Autodesk Fusion 360 part; units mm, degrees
(part 5 of 5)
sketch "Sketch4" plane through (0, 0, 0) normal (0, 0, -1) x (1, 0, 0)
  spline S0 degree 3 poles (245.0152, -3.6397) (245.0152, -3.0095) (244.82, -2.6944) (244.4293, -2.6944) knots -1 -1 -1 -1 0 0 0 0
  spline S1 degree 3 poles (244.2163, -5.1842) (244.7489, -4.6693) (245.0152, -4.1546) (245.0152, -3.6397) knots -1 -1 -1 -1 0 0 0 0
  spline S2 degree 3 poles (243.9766, -3.2536) (243.9766, -3.2625) (244.0565, -3.906) (244.2163, -5.1842) knots -1 -1 -1 -1 0 0 0 0
  spline S3 degree 3 poles (244.4293, -2.6944) (244.1277, -2.6944) (243.9766, -2.8808) (243.9766, -3.2536) knots -1 -1 -1 -1 0 0 0 0
  spline S4 degree 3 poles (271.6477, -6.9285) (271.8784, -6.9285) (272.1314, -6.8752) (272.4066, -6.7687) knots -1 -1 -1 -1 0 0 0 0
  spline S5 degree 3 poles (270.2896, -6.276) (270.6268, -6.711) (271.0795, -6.9285) (271.6477, -6.9285) knots -1 -1 -1 -1 0 0 0 0
  spline S6 degree 3 poles (269.7037, -4.3587) (269.7657, -5.2109) (269.9611, -5.85) (270.2896, -6.276) knots -1 -1 -1 -1 0 0 0 0
  spline S7 degree 3 poles (269.6904, -4.1324) (269.6904, -4.2033) (269.6948, -4.2788) (269.7037, -4.3587) knots -1 -1 -1 -1 0 0 0 0
  spline S8 degree 3 poles (269.9967, -3.0938) (269.7924, -3.3512) (269.6904, -3.6973) (269.6904, -4.1324) knots -1 -1 -1 -1 0 0 0 0
  spline S9 degree 3 poles (270.8089, -2.7077) (270.4804, -2.7077) (270.2097, -2.8365) (269.9967, -3.0938) knots -1 -1 -1 -1 0 0 0 0
  spline S10 degree 3 poles (272.0738, -3.8794) (271.7896, -3.0982) (271.3681, -2.7077) (270.8089, -2.7077) knots -1 -1 -1 -1 0 0 0 0
  line L0 (272.0738, -3.8794) -> (272.4066, -6.7687)
  spline S11 degree 3 poles (249.2375, -3.3867) (249.2375, -3.5998) (249.2951, -4.1546) (249.4106, -5.0511) knots -1 -1 -1 -1 0 0 0 0
  spline S12 degree 3 poles (249.4638, -2.8675) (249.313, -3.0095) (249.2375, -3.1826) (249.2375, -3.3867) knots -1 -1 -1 -1 0 0 0 0
  spline S13 degree 3 poles (250.1162, -2.6677) (249.841, -2.6677) (249.6236, -2.7343) (249.4638, -2.8675) knots -1 -1 -1 -1 0 0 0 0
  spline S14 degree 3 poles (251.2347, -3.2935) (250.9418, -2.8764) (250.5689, -2.6677) (250.1162, -2.6677) knots -1 -1 -1 -1 0 0 0 0
  spline S15 degree 3 poles (251.7673, -5.2641) (251.7673, -4.4563) (251.5898, -3.7995) (251.2347, -3.2935) knots -1 -1 -1 -1 0 0 0 0
  spline S16 degree 3 poles (251.501, -6.3027) (251.6784, -6.0008) (251.7673, -5.6546) (251.7673, -5.2641) knots -1 -1 -1 -1 0 0 0 0
  spline S17 degree 3 poles (250.6755, -6.7554) (251.0483, -6.7554) (251.3235, -6.6045) (251.501, -6.3027) knots -1 -1 -1 -1 0 0 0 0
  spline S18 degree 3 poles (249.5171, -5.85) (249.7834, -6.4536) (250.1695, -6.7554) (250.6755, -6.7554) knots -1 -1 -1 -1 0 0 0 0
  line L1 (249.5171, -5.85) -> (249.4106, -5.0511)
  spline S19 degree 3 poles (270.0499, 0.4346) (270.0499, -0.311) (270.6402, -1.0344) (271.8208, -1.7357) knots -1 -1 -1 -1 0 0 0 0
  spline S20 degree 3 poles (270.2496, 0.9938) (270.1165, 0.8607) (270.0499, 0.6743) (270.0499, 0.4346) knots -1 -1 -1 -1 0 0 0 0
  spline S21 degree 3 poles (270.729, 1.2068) (270.5513, 1.2068) (270.3915, 1.1359) (270.2496, 0.9938) knots -1 -1 -1 -1 0 0 0 0
  spline S22 degree 3 poles (271.5944, 0.2615) (271.5145, 0.8917) (271.226, 1.2068) (270.729, 1.2068) knots -1 -1 -1 -1 0 0 0 0
  line L2 (271.5944, 0.2615) -> (271.8208, -1.7357)
  spline S23 degree 3 poles (254.5822, -2.0872) (254.0928, -2.1577) (253.5454, -2.2239) (253.0284, -2.2637) knots 0.397503 0.397503 0.397503 0.397503 1 1 1 1
  spline S24 degree 3 poles (253.0284, -2.2637) (252.7959, -2.2817) (252.5688, -2.2944) (252.3554, -2.2998) knots 0 0 0 0 0.530693 0.530693 0.530693 0.530693
  spline S25 degree 3 poles (252.3554, -2.2998) (251.6864, -1.7551) (250.829, -1.4827) (249.7834, -1.4827) knots 0.050062 0.050062 0.050062 0.050062 1 1 1 1
  spline S26 degree 3 poles (249.7834, -1.4827) (249.3396, -1.5004) (248.9535, -1.5803) (248.625, -1.7224) knots 0 0 0 0 1 1 1 1
  spline S27 degree 3 poles (248.625, -1.7224) (248.2965, -1.8645) (248.0525, -2.0419) (247.8927, -2.255) knots 0 0 0 0 1 1 1 1
  spline S28 degree 3 poles (247.8927, -2.255) (247.6718, -2.5408) (247.5317, -2.8028) (247.4725, -3.0411) knots 0 0 0 0 0.731862 0.731862 0.731862 0.731862
  spline S29 degree 3 poles (247.4725, -3.0411) (247.287, -3.1929) (247.0989, -3.2785) (246.9137, -3.3116) knots 0.13739 0.13739 0.13739 0.13739 1 1 1 1
  spline S30 degree 3 poles (246.9137, -3.3116) (246.6993, -3.35) (246.4954, -3.3167) (246.3122, -3.2441) knots 0 0 0 0 1 1 1 1
  spline S31 degree 3 poles (246.3122, -3.2441) (246.1226, -3.1688) (245.953, -3.0508) (245.812, -2.9222) knots 0 0 0 0 0.743467 0.743467 0.743467 0.743467
  spline S32 degree 3 poles (245.812, -2.9222) (245.7256, -2.5498) (245.5577, -2.2475) (245.3081, -2.0153) knots 0.346286 0.346286 0.346286 0.346286 1 1 1 1
  spline S33 degree 3 poles (245.3081, -2.0153) (244.9265, -1.6602) (244.4472, -1.4827) (243.8701, -1.4827) knots 0 0 0 0 1 1 1 1
  spline S34 degree 3 poles (243.8701, -1.4827) (243.2932, -1.4827) (242.8715, -1.6602) (242.6052, -2.0153) knots 0 0 0 0 1 1 1 1
  spline S35 degree 3 poles (242.6052, -2.0153) (242.357, -2.3545) (242.2244, -2.7749) (242.2076, -3.2761) knots 0 0 0 0 0.932227 0.932227 0.932227 0.932227
  spline S36 degree 3 poles (242.2076, -3.2761) (241.9882, -3.027) (241.7354, -2.7798) (241.4493, -2.5346) knots 0.616308 0.616308 0.616308 0.616308 1 1 1 1
  spline S37 degree 3 poles (241.4493, -2.5346) (241.0765, -2.224) (240.6327, -1.971) (240.1178, -1.7757) knots 0 0 0 0 1 1 1 1
  spline S38 degree 3 poles (240.1178, -1.7757) (239.6119, -1.5803) (239.0882, -1.4827) (238.5467, -1.4827) knots 0 0 0 0 1 1 1 1
  spline S39 degree 3 poles (238.5467, -1.4827) (237.659, -1.4827) (236.9578, -1.7534) (236.4429, -2.2949) knots 0 0 0 0 1 1 1 1
  spline S40 degree 3 poles (236.4429, -2.2949) (235.8938, -2.8795) (235.6187, -3.6274) (235.6174, -4.5389) knots 0 0 0 0 0.99774 0.99774 0.99774 0.99774
  spline S41 degree 3 poles (235.6174, -4.5389) (235.515, -4.5909) (235.4125, -4.6249) (235.3108, -4.6431) knots 0.526695 0.526695 0.526695 0.526695 1 1 1 1
  spline S42 degree 3 poles (235.3108, -4.6431) (235.0964, -4.6815) (234.8926, -4.6482) (234.7093, -4.5756) knots 0 0 0 0 1 1 1 1
  spline S43 degree 3 poles (234.7093, -4.5756) (234.6486, -4.5514) (234.5899, -4.5229) (234.5335, -4.4911) knots 0 0 0 0 0.23829 0.23829 0.23829 0.23829
  spline S44 degree 3 poles (234.5335, -4.4911) (234.3844, -3.9886) (234.2169, -3.5717) (234.031, -3.2403) knots 0.544726 0.544726 0.544726 0.544726 1 1 1 1
  spline S45 degree 3 poles (234.031, -3.2403) (233.8446, -2.9297) (233.6316, -2.6322) (233.3919, -2.3482) knots 0 0 0 0 1 1 1 1
  spline S46 degree 3 poles (233.3919, -2.3482) (232.8948, -1.7713) (232.198, -1.4827) (231.3015, -1.4827) knots 0 0 0 0 1 1 1 1
  spline S47 degree 3 poles (231.3015, -1.4827) (230.4138, -1.4827) (229.7792, -1.8645) (229.3975, -2.6278) knots 0 0 0 0 1 1 1 1
  spline S48 degree 3 poles (229.3975, -2.6278) (228.9093, -1.8645) (228.1681, -1.4827) (227.1739, -1.4827) knots 0 0 0 0 1 1 1 1
  spline S49 degree 3 poles (227.1739, -1.4827) (226.5348, -1.4827) (226.0377, -1.6648) (225.6827, -2.0286) knots 0 0 0 0 1 1 1 1
  spline S50 degree 3 poles (225.6827, -2.0286) (225.3365, -2.4014) (225.1634, -2.8941) (225.1634, -3.5066) knots 0 0 0 0 1 1 1 1
  spline S51 degree 3 poles (225.1634, -3.5066) (225.1634, -3.5865) (225.1723, -3.7063) (225.19, -3.8661) knots 0 0 0 0 1 1 1 1
  line L3 (225.19, -3.8661) -> (225.6827, -7.6208)
  spline S52 degree 3 poles (225.6827, -7.6208) (224.7329, -8.3043) (224.258, -9.0721) (224.258, -9.9243) knots 0 0 0 0 1 1 1 1
  spline S53 degree 3 poles (224.258, -9.9243) (224.258, -10.4658) (224.4444, -10.8963) (224.8172, -11.2158) knots 0 0 0 0 1 1 1 1
  spline S54 degree 3 poles (224.8172, -11.2158) (225.19, -11.5354) (225.6427, -11.6952) (226.1753, -11.6952) knots 0 0 0 0 1 1 1 1
  spline S55 degree 3 poles (226.1753, -11.6952) (227.3381, -11.6952) (227.9195, -11.1182) (227.9195, -9.9642) knots 0 0 0 0 1 1 1 1
  spline S56 degree 3 poles (227.9195, -9.9642) (227.9195, -9.9465) (227.9151, -9.9243) (227.9062, -9.8977) knots 0 0 0 0 1 1 1 1
  spline S57 degree 3 poles (227.9062, -9.8977) (227.9062, -9.871) (227.9018, -9.8267) (227.8929, -9.7645) knots 0 0 0 0 1 1 1 1
  spline S58 degree 3 poles (227.8929, -9.7645) (227.8929, -9.7113) (227.884, -9.6447) (227.8663, -9.5648) knots 0 0 0 0 1 1 1 1
  spline S59 degree 3 poles (227.8663, -9.5648) (227.8574, -9.4938) (227.8396, -9.3828) (227.813, -9.2319) knots 0 0 0 0 1 1 1 1
  spline S60 degree 3 poles (227.813, -9.2319) (227.7953, -9.081) (227.7731, -8.9124) (227.7464, -8.726) knots 0 0 0 0 1 1 1 1
  spline S61 degree 3 poles (227.7464, -8.726) (227.7198, -8.5484) (227.6843, -8.3088) (227.6399, -8.007) knots 0 0 0 0 1 1 1 1
  spline S62 degree 3 poles (227.6399, -8.007) (227.5955, -7.7052) (227.5467, -7.3767) (227.4935, -7.0217) knots 0 0 0 0 1 1 1 1
  spline S63 degree 3 poles (227.4935, -7.0217) (227.4491, -6.6755) (227.3914, -6.2494) (227.3204, -5.7434) knots 0 0 0 0 1 1 1 1
  spline S64 degree 3 poles (227.3204, -5.7434) (227.2494, -5.2375) (227.1872, -4.807) (227.134, -4.4519) knots 0 0 0 0 1 1 1 1
  spline S65 degree 3 poles (227.134, -4.4519) (227.0807, -4.0968) (227.0541, -3.8394) (227.0541, -3.6797) knots 0 0 0 0 1 1 1 1
  spline S66 degree 3 poles (227.0541, -3.6797) (227.0541, -3.0849) (227.2849, -2.7876) (227.7464, -2.7876) knots 0 0 0 0 1 1 1 1
  spline S67 degree 3 poles (227.7464, -2.7876) (228.3855, -2.7876) (228.7806, -3.369) (228.9314, -4.5318) knots 0 0 0 0 1 1 1 1
  line L4 (228.9314, -4.5318) -> (229.7836, -11.2558)
  spline S68 degree 3 poles (229.7836, -11.2558) (230.0765, -11.3889) (230.4271, -11.4555) (230.8355, -11.4555) knots 0 0 0 0 1 1 1 1
  spline S69 degree 3 poles (230.8355, -11.4555) (231.4036, -11.4555) (231.6876, -11.2336) (231.6876, -10.7897) knots 0 0 0 0 1 1 1 1
  line L5 (231.6876, -10.7897) -> (231.6743, -10.6167)
  spline S70 degree 3 poles (231.6743, -10.6167) (231.337, -8.0247) (231.1151, -6.4269) (231.0085, -5.8233) knots 0 0 0 0 1 1 1 1
  spline S71 degree 3 poles (231.0085, -5.8233) (230.831, -4.8291) (230.7423, -4.0702) (230.7423, -3.5465) knots 0 0 0 0 1 1 1 1
  spline S72 degree 3 poles (230.7423, -3.5465) (230.7423, -3.0316) (230.9642, -2.7743) (231.408, -2.7743) knots 0 0 0 0 1 1 1 1
  spline S73 degree 3 poles (231.408, -2.7743) (231.7808, -2.7743) (232.1137, -3.0406) (232.4066, -3.5731) knots 0 0 0 0 1 1 1 1
  spline S74 degree 3 poles (232.4066, -3.5731) (232.6995, -4.1147) (232.9214, -4.7848) (233.0723, -5.5837) knots 0 0 0 0 1 1 1 1
  spline S75 degree 3 poles (233.0723, -5.5837) (233.383, -7.2525) (233.5383, -8.6949) (233.5383, -9.911) knots 0 0 0 0 1 1 1 1
  spline S76 degree 3 poles (233.5383, -9.911) (233.5383, -10.4791) (233.4895, -10.9717) (233.3919, -11.3889) knots 0 0 0 0 1 1 1 1
  spline S77 degree 3 poles (233.3919, -11.3889) (233.747, -11.6019) (234.173, -11.7085) (234.6701, -11.7085) knots 0 0 0 0 1 1 1 1
  spline S78 degree 3 poles (234.6701, -11.7085) (235.1672, -11.7085) (235.4157, -11.4155) (235.4157, -10.8297) knots 0 0 0 0 1 1 1 1
  spline S79 degree 3 poles (235.4157, -10.8297) (235.4157, -9.9154) (235.2737, -8.5262) (234.9897, -6.6622) knots 0 0 0 0 1 1 1 1
  spline S80 degree 3 poles (234.9897, -6.6622) (234.9205, -6.1966) (234.8433, -5.768) (234.7582, -5.3766) knots 0 0 0 0 0.299729 0.299729 0.299729 0.299729
  spline S81 degree 3 poles (234.7582, -5.3766) (234.8814, -5.3921) (235.0075, -5.416) (235.1323, -5.4454) knots 0.430322 0.430322 0.430322 0.430322 1 1 1 1
  spline S82 degree 3 poles (235.1323, -5.4454) (235.3655, -5.5005) (235.5978, -5.5756) (235.8043, -5.6532) knots 0 0 0 0 0.607186 0.607186 0.607186 0.607186
  spline S83 degree 3 poles (235.8043, -5.6532) (235.9716, -6.1206) (236.251, -6.5502) (236.6427, -6.9418) knots 0.426984 0.426984 0.426984 0.426984 1 1 1 1
  spline S84 degree 3 poles (236.6427, -6.9418) (237.335, -7.6253) (238.1605, -7.967) (239.1192, -7.967) knots 0 0 0 0 1 1 1 1
  spline S85 degree 3 poles (239.1192, -7.967) (239.8026, -7.967) (240.3575, -7.8161) (240.7836, -7.5143) knots 0 0 0 0 1 1 1 1
  spline S86 degree 3 poles (240.7836, -7.5143) (241.2096, -7.2214) (241.427, -6.822) (241.436, -6.316) knots 0 0 0 0 1 1 1 1
  spline S87 degree 3 poles (241.436, -6.316) (241.436, -5.6326) (241.1607, -5.0777) (240.6105, -4.6516) knots 0 0 0 0 1 1 1 1
  spline S88 degree 3 poles (240.6105, -4.6516) (240.0689, -4.2256) (239.3233, -3.9283) (238.3736, -3.7595) knots 0 0 0 0 1 1 1 1
  line L6 (238.3736, -3.7595) -> (238.1872, -4.5451)
  spline S89 degree 3 poles (238.1872, -4.5451) (238.7375, -4.6606) (239.1458, -4.8824) (239.4121, -5.2109) knots 0 0 0 0 1 1 1 1
  spline S90 degree 3 poles (239.4121, -5.2109) (239.6874, -5.5393) (239.8249, -5.8543) (239.8249, -6.1562) knots 0 0 0 0 1 1 1 1
  spline S91 degree 3 poles (239.8249, -6.1562) (239.8249, -6.4669) (239.7406, -6.6755) (239.5719, -6.782) knots 0 0 0 0 1 1 1 1
  spline S92 degree 3 poles (239.5719, -6.782) (239.4121, -6.8974) (239.2347, -6.9551) (239.0393, -6.9551) knots 0 0 0 0 1 1 1 1
  spline S93 degree 3 poles (239.0393, -6.9551) (238.6221, -6.9551) (238.2537, -6.7199) (237.9342, -6.2494) knots 0 0 0 0 1 1 1 1
  spline S94 degree 3 poles (237.9342, -6.2494) (237.6235, -5.7878) (237.4682, -5.2331) (237.4682, -4.5851) knots 0 0 0 0 1 1 1 1
  spline S95 degree 3 poles (237.4682, -4.5851) (237.4682, -3.946) (237.6191, -3.4666) (237.9209, -3.1471) knots 0 0 0 0 1 1 1 1
  spline S96 degree 3 poles (237.9209, -3.1471) (238.2315, -2.8365) (238.6132, -2.6811) (239.066, -2.6811) knots 0 0 0 0 1 1 1 1
  spline S97 degree 3 poles (239.066, -2.6811) (239.7317, -2.6811) (240.3708, -2.9118) (240.9833, -3.3734) knots 0 0 0 0 1 1 1 1
  spline S98 degree 3 poles (240.9833, -3.3734) (241.535, -3.7893) (241.9931, -4.3203) (242.3576, -4.9667) knots 0 0 0 0 0.900867 0.900867 0.900867 0.900867
  line L7 (242.3576, -4.9667) -> (242.6851, -7.8206)
  spline S99 degree 3 poles (242.6851, -7.8206) (243.0047, -7.9182) (243.3288, -7.967) (243.6571, -7.967) knots 0 0 0 0 1 1 1 1
  spline S100 degree 3 poles (243.6571, -7.967) (244.1986, -7.967) (244.4693, -7.7673) (244.4693, -7.3679) knots 0 0 0 0 1 1 1 1
  line L8 (244.4693, -7.3679) -> (244.4693, -7.3412)
  spline S101 degree 3 poles (244.4693, -7.3412) (244.8244, -7.7584) (245.2771, -7.967) (245.8274, -7.967) knots 0 0 0 0 1 1 1 1
  spline S102 degree 3 poles (245.8274, -7.967) (246.2268, -7.967) (246.5376, -7.8738) (246.7594, -7.6874) knots 0 0 0 0 1 1 1 1
  spline S103 degree 3 poles (246.7594, -7.6874) (246.9814, -7.5099) (247.0923, -7.2702) (247.0923, -6.9684) knots 0 0 0 0 1 1 1 1
  spline S104 degree 3 poles (247.0923, -6.9684) (247.0923, -6.6666) (246.977, -6.4181) (246.7461, -6.2228) knots 0 0 0 0 1 1 1 1
  spline S105 degree 3 poles (246.7461, -6.2228) (246.5243, -6.0364) (246.2314, -5.9432) (245.8673, -5.9432) knots 0 0 0 0 1 1 1 1
  line L9 (245.8673, -5.9432) -> (245.8141, -5.9432)
  spline S106 degree 3 poles (245.8141, -5.9432) (245.8319, -6.0407) (245.8407, -6.1339) (245.8407, -6.2228) knots 0 0 0 0 1 1 1 1
  spline S107 degree 3 poles (245.8407, -6.2228) (245.8407, -6.6134) (245.6588, -6.8086) (245.2948, -6.8086) knots 0 0 0 0 1 1 1 1
  spline S108 degree 3 poles (245.2948, -6.8086) (244.9399, -6.8086) (244.6557, -6.5779) (244.4426, -6.1163) knots 0 0 0 0 1 1 1 1
  spline S109 degree 3 poles (244.4426, -6.1163) (245.2391, -5.4893) (245.7047, -4.7982) (245.8395, -4.0427) knots 0 0 0 0 0.830833 0.830833 0.830833 0.830833
  spline S110 degree 3 poles (245.8395, -4.0427) (245.9193, -4.0302) (246.003, -4.0252) (246.0883, -4.0258) knots 0.414198 0.414198 0.414198 0.414198 1 1 1 1
  spline S111 degree 3 poles (246.0883, -4.0258) (246.2932, -4.0276) (246.5161, -4.0624) (246.7351, -4.1139) knots 0 0 0 0 1 1 1 1
  spline S112 degree 3 poles (246.7351, -4.1139) (247.0125, -4.1794) (247.2885, -4.2732) (247.5216, -4.366) knots 0 0 0 0 0.722113 0.722113 0.722113 0.722113
  spline S113 degree 3 poles (247.5216, -4.366) (247.5367, -4.4968) (247.5538, -4.6364) (247.5731, -4.7848) knots 0.782884 0.782884 0.782884 0.782884 1 1 1 1
  spline S114 degree 3 poles (247.5731, -4.7848) (247.7595, -6.1872) (248.0258, -8.4552) (248.372, -11.5886) knots 0 0 0 0 1 1 1 1
  spline S115 degree 3 poles (248.372, -11.5886) (248.5584, -11.6596) (248.807, -11.6952) (249.1176, -11.6952) knots 0 0 0 0 1 1 1 1
  spline S116 degree 3 poles (249.1176, -11.6952) (249.8277, -11.6952) (250.1828, -11.491) (250.1828, -11.0827) knots 0 0 0 0 1 1 1 1
  line L10 (250.1828, -11.0827) -> (249.7301, -7.541)
  spline S117 degree 3 poles (249.7301, -7.541) (250.1472, -7.8339) (250.6711, -7.9803) (251.3013, -7.9803) knots 0 0 0 0 1 1 1 1
  spline S118 degree 3 poles (251.3013, -7.9803) (251.9404, -7.9803) (252.4906, -7.7185) (252.9523, -7.1948) knots 0 0 0 0 1 1 1 1
  spline S119 degree 3 poles (252.9523, -7.1948) (253.4139, -6.6711) (253.6446, -6.0586) (253.6446, -5.3573) knots 0 0 0 0 1 1 1 1
  spline S120 degree 3 poles (253.6446, -5.3573) (253.6446, -5.2597) (253.6403, -5.1576) (253.6313, -5.0511) knots 0 0 0 0 1 1 1 1
  spline S121 degree 3 poles (253.6313, -5.0511) (253.5646, -4.2555) (253.3606, -3.5887) (253.0195, -3.0507) knots 0 0 0 0 0.684208 0.684208 0.684208 0.684208
  spline S122 degree 3 poles (253.0195, -3.0507) (253.1893, -2.9872) (253.3743, -2.9283) (253.571, -2.877) knots 0.64979 0.64979 0.64979 0.64979 1 1 1 1
  spline S123 degree 3 poles (253.571, -2.877) (253.7786, -2.8228) (254, -2.7769) (254.2316, -2.7427) knots 0 0 0 0 0.33927 0.33927 0.33927 0.33927
  spline S124 degree 3 poles (254.2316, -2.7427) (254.1928, -2.8932) (254.1734, -3.0546) (254.1734, -3.227) knots 0.665214 0.665214 0.665214 0.665214 1 1 1 1
  spline S125 degree 3 poles (254.1734, -3.227) (254.1734, -3.3512) (254.1957, -3.5688) (254.24, -3.8794) knots 0 0 0 0 1 1 1 1
  spline S126 degree 3 poles (254.24, -3.8794) (254.4443, -5.5304) (254.5995, -6.8442) (254.706, -7.8206) knots 0 0 0 0 1 1 1 1
  spline S127 degree 3 poles (254.706, -7.8206) (254.9813, -7.9182) (255.2342, -7.967) (255.465, -7.967) knots 0 0 0 0 1 1 1 1
  spline S128 degree 3 poles (255.465, -7.967) (255.6959, -7.967) (255.869, -7.9581) (255.9842, -7.9404) knots 0 0 0 0 1 1 1 1
  spline S129 degree 3 poles (255.9842, -7.9404) (256.0997, -7.9226) (256.2106, -7.8561) (256.3171, -7.7407) knots 0 0 0 0 1 1 1 1
  spline S130 degree 3 poles (256.3171, -7.7407) (256.4236, -7.6253) (256.4769, -7.4611) (256.4769, -7.248) knots 0 0 0 0 1 1 1 1
  line L11 (256.4769, -7.248) -> (256.0375, -3.8528)
  spline S131 degree 3 poles (256.0375, -3.8528) (256.0198, -3.7462) (256.0109, -3.6487) (256.0109, -3.5598) knots 0 0 0 0 1 1 1 1
  spline S132 degree 3 poles (256.0109, -3.5598) (256.0109, -3.0362) (256.2505, -2.7743) (256.7299, -2.7743) knots 0 0 0 0 1 1 1 1
  spline S133 degree 3 poles (256.7299, -2.7743) (257.1738, -2.7743) (257.5421, -2.9917) (257.835, -3.4267) knots 0 0 0 0 1 1 1 1
  spline S134 degree 3 poles (257.835, -3.4267) (257.835, -3.5243) (257.8439, -3.6797) (257.8616, -3.8927) knots 0 0 0 0 1 1 1 1
  line L12 (257.8616, -3.8927) -> (258.301, -7.4344)
  spline S135 degree 3 poles (258.301, -7.4344) (258.3632, -7.5853) (258.4963, -7.7096) (258.7004, -7.8072) knots 0 0 0 0 1 1 1 1
  spline S136 degree 3 poles (258.7004, -7.8072) (258.9047, -7.9138) (259.1577, -7.967) (259.4594, -7.967) knots 0 0 0 0 1 1 1 1
  spline S137 degree 3 poles (259.4594, -7.967) (259.7702, -7.967) (260.0009, -7.9226) (260.1517, -7.8339) knots 0 0 0 0 1 1 1 1
  spline S138 degree 3 poles (260.1517, -7.8339) (259.7879, -4.9579) (259.6058, -3.4267) (259.6058, -3.2403) knots 0 0 0 0 1 1 1 1
  spline S139 degree 3 poles (259.6058, -3.2403) (259.6058, -2.8852) (259.7346, -2.7077) (259.992, -2.7077) knots 0 0 0 0 1 1 1 1
  spline S140 degree 3 poles (259.992, -2.7077) (260.2229, -2.7077) (260.4713, -2.8631) (260.7376, -3.1737) knots 0 0 0 0 1 1 1 1
  spline S141 degree 3 poles (260.7376, -3.1737) (260.8786, -3.3374) (261.0044, -3.5419) (261.1151, -3.7872) knots 0 0 0 0 0.512298 0.512298 0.512298 0.512298
  line L13 (261.1151, -3.7872) -> (261.5876, -7.8339)
  spline S142 degree 3 poles (261.5876, -7.8339) (261.9605, -7.9315) (262.2444, -7.9803) (262.4398, -7.9803) knots 0 0 0 0 1 1 1 1
  spline S143 degree 3 poles (262.4398, -7.9803) (263.0344, -7.9803) (263.3452, -7.7629) (263.3718, -7.3279) knots 0 0 0 0 1 1 1 1
  spline S144 degree 3 poles (263.3718, -7.3279) (263.8066, -7.754) (264.3259, -7.967) (264.9296, -7.967) knots 0 0 0 0 1 1 1 1
  spline S145 degree 3 poles (264.9296, -7.967) (265.5421, -7.967) (266.0215, -7.8161) (266.3676, -7.5143) knots 0 0 0 0 1 1 1 1
  spline S146 degree 3 poles (266.3676, -7.5143) (266.7138, -7.2125) (266.8869, -6.8308) (266.8869, -6.3693) knots 0 0 0 0 1 1 1 1
  spline S147 degree 3 poles (266.8869, -6.3693) (266.8869, -6.245) (266.8603, -6.0097) (266.807, -5.6636) knots 0 0 0 0 1 1 1 1
  spline S148 degree 3 poles (266.807, -5.6636) (266.6027, -4.3144) (266.5008, -3.5288) (266.5008, -3.3068) knots 0 0 0 0 1 1 1 1
  spline S149 degree 3 poles (266.5008, -3.3068) (266.5008, -2.8985) (266.6383, -2.6944) (266.9135, -2.6944) knots 0 0 0 0 1 1 1 1
  spline S150 degree 3 poles (266.9135, -2.6944) (267.2996, -2.6944) (267.6257, -2.9522) (267.892, -3.4679) knots 0 0 0 0 0.639657 0.639657 0.639657 0.639657
  spline S151 degree 3 poles (267.892, -3.4679) (267.8482, -3.6797) (267.8264, -3.9056) (267.8264, -4.1457) knots 0.689137 0.689137 0.689137 0.689137 1 1 1 1
  spline S152 degree 3 poles (267.8264, -4.1457) (267.8264, -5.3084) (268.168, -6.2361) (268.8516, -6.9285) knots 0 0 0 0 1 1 1 1
  spline S153 degree 3 poles (268.8516, -6.9285) (269.535, -7.6208) (270.4005, -7.967) (271.448, -7.967) knots 0 0 0 0 1 1 1 1
  spline S154 degree 3 poles (271.448, -7.967) (271.9361, -7.967) (272.3844, -7.8871) (272.7928, -7.7274) knots 0 0 0 0 1 1 1 1
  spline S155 degree 3 poles (272.7928, -7.7274) (273.0678, -7.896) (273.3564, -7.9803) (273.6582, -7.9803) knots 0 0 0 0 1 1 1 1
  spline S156 degree 3 poles (273.6582, -7.9803) (273.9599, -7.9803) (274.1996, -7.9404) (274.3772, -7.8605) knots 0 0 0 0 1 1 1 1
  line L14 (274.3772, -7.8605) -> (273.8979, -4.1057)
  spline S157 degree 3 poles (273.8979, -4.1057) (274.5547, -4.6117) (275.0517, -5.0733) (275.3891, -5.4905) knots 0 0 0 0 1 1 1 1
  line L15 (275.3891, -5.4905) -> (275.7753, -4.6783)
  spline S158 degree 3 poles (275.7753, -4.6783) (275.2693, -4.1457) (274.5946, -3.5775) (273.7514, -2.974) knots 0 0 0 0 1 1 1 1
  line L16 (273.7514, -2.974) -> (273.3919, -0.1912)
  spline S159 degree 3 poles (273.3919, -0.1912) (273.2942, 0.6433) (273.0191, 1.2824) (272.5664, 1.7261) knots 0 0 0 0 1 1 1 1
  spline S160 degree 3 poles (272.5664, 1.7261) (272.1225, 2.1788) (271.5456, 2.4052) (270.8355, 2.4052) knots 0 0 0 0 1 1 1 1
  spline S161 degree 3 poles (270.8355, 2.4052) (270.4271, 2.4052) (270.0277, 2.272) (269.6372, 2.0057) knots 0 0 0 0 1 1 1 1
  spline S162 degree 3 poles (269.6372, 2.0057) (269.2288, 1.7217) (269.0247, 1.2645) (269.0247, 0.6343) knots 0 0 0 0 1 1 1 1
  spline S163 degree 3 poles (269.0247, 0.6343) (269.0247, -0.1379) (269.3929, -0.8436) (270.1298, -1.4827) knots 0 0 0 0 1 1 1 1
  spline S164 degree 3 poles (270.1298, -1.4827) (269.4995, -1.527) (268.9581, -1.789) (268.5054, -2.2683) knots 0 0 0 0 1 1 1 1
  spline S165 degree 3 poles (268.5054, -2.2683) (268.4184, -2.3605) (268.3397, -2.4581) (268.2694, -2.5611) knots 0 0 0 0 0.192295 0.192295 0.192295 0.192295
  spline S166 degree 3 poles (268.2694, -2.5611) (267.7992, -1.8422) (267.1697, -1.4827) (266.381, -1.4827) knots 0.321658 0.321658 0.321658 0.321658 1 1 1 1
  spline S167 degree 3 poles (266.381, -1.4827) (265.8305, -1.4827) (265.4223, -1.6514) (265.156, -1.9887) knots 0 0 0 0 1 1 1 1
  spline S168 degree 3 poles (265.156, -1.9887) (264.8897, -2.3259) (264.7566, -2.6811) (264.7566, -3.0539) knots 0 0 0 0 1 1 1 1
  line L17 (264.7566, -3.0539) -> (265.0761, -6.0231)
  spline S169 degree 3 poles (265.0761, -6.0231) (265.0761, -6.2627) (265.0139, -6.4625) (264.8897, -6.6222) knots 0 0 0 0 1 1 1 1
  spline S170 degree 3 poles (264.8897, -6.6222) (264.7653, -6.782) (264.5568, -6.8619) (264.2639, -6.8619) knots 0 0 0 0 1 1 1 1
  spline S171 degree 3 poles (264.2639, -6.8619) (263.9797, -6.8619) (263.7357, -6.7332) (263.5316, -6.4758) knots 0 0 0 0 1 1 1 1
  spline S172 degree 3 poles (263.5316, -6.4758) (263.3363, -6.2271) (263.212, -5.9122) (263.1588, -5.5304) knots 0 0 0 0 1 1 1 1
  spline S173 degree 3 poles (263.1588, -5.5304) (262.8392, -3.0982) (262.6705, -1.7757) (262.6528, -1.5626) knots 0 0 0 0 1 1 1 1
  line L18 (262.6528, -1.5626) -> (260.8553, -1.5626)
  line L19 (260.8553, -1.5626) -> (260.9056, -1.9933)
  spline S174 degree 3 poles (260.9056, -1.9933) (260.476, -1.6617) (260.0339, -1.496) (259.5792, -1.496) knots 0.033773 0.033773 0.033773 0.033773 1 1 1 1
  spline S175 degree 3 poles (259.5792, -1.496) (258.807, -1.496) (258.2877, -1.7933) (258.0214, -2.3881) knots 0 0 0 0 1 1 1 1
  spline S176 degree 3 poles (258.0214, -2.3881) (257.5599, -1.7933) (256.9429, -1.496) (256.1706, -1.496) knots 0 0 0 0 1 1 1 1
  spline S177 degree 3 poles (256.1706, -1.496) (255.5315, -1.496) (255.0389, -1.6558) (254.6927, -1.9754) knots 0 0 0 0 1 1 1 1
  spline S178 degree 3 poles (254.6927, -1.9754) (254.6537, -2.0114) (254.6168, -2.0487) (254.5822, -2.0872) knots 0 0 0 0 0.112782 0.112782 0.112782 0.112782
  line L20 (213.8586, 6.0554) -> (286.7595, 6.0554)
  line L21 (286.7595, 6.0554) -> (286.7595, -29.9009)
  line L22 (286.7595, -29.9009) -> (213.8586, -29.9009)
  line L23 (213.8586, -29.9009) -> (213.8586, 6.0554)
  line L24 (302.4222, 30.8643) -> (309.9222, 30.8643)
  line L25 (309.9222, 30.8643) -> (309.9222, 23.3643)
  line L26 (309.9222, 23.3643) -> (302.4222, 23.3643)
  line L27 (302.4222, 23.3643) -> (302.4222, 30.8643)
  line L28 (212.8586, -30.9009) -> (287.7595, -30.9009)
  line L29 (287.7595, -30.9009) -> (287.7595, 7.0554)
  line L30 (287.7595, 7.0554) -> (212.8586, 7.0554)
  line L31 (212.8586, 7.0554) -> (212.8586, -30.9009)
  dimension "d13" = 7.5
  dimension "d14" = 7.5
  dimension "d15" = 1
  dimension "d16" = 1
  dimension "d18" = 1
  dimension "d19" = 1
  constraint horizontal L20
  constraint vertical L21
  constraint horizontal L22
  constraint vertical L23
  constraint horizontal L24
  constraint vertical L25
  constraint horizontal L26
  constraint vertical L27
  constraint horizontal L28
  constraint vertical L29
  constraint horizontal L30
  constraint vertical L31
  measures "d13" distance of L24.start L24.end
  measures "d14" distance of L24.start L26.end
  measures "d15" distance of L22 L28
  measures "d16" distance of L23 L31
  measures "d18" distance of L21 L29
  measures "d19" distance of L20 L30
extrude "Extrude4" add sketch "Sketch4" along normal blind 0.4 contours S0 S1 S2 S3 | S4 S5 S6 S7 S8 S9 S10 L0 | S11 S12 S13 S14 S15 S16 S17 S18 L1 | S19 S20 S21 S22 L2 | S23 S24 S25 S26 S27 S28 S29 S30 S31 S32 S33 S34 S35 S36 S37 S38 S39 S40 S41 S42 S43 S44 S45 S46 S47 S48 S49 S50 S51 L3 S52 S53 S54 S55 S56 S57 S58 S59 S60 S61 S62 S63 S64 S65 S66 S67 L4 S68 S69 L5 S70 S71 S72 S73 S74 S75 S76 S77 S78 S79 S80 S81 S82 S83 S84 S85 S86 S87 S88 L6 S89 S90 S91 S92 S93 S94 S95 S96 S97 S98 L7 S99 S100 L8 S101 S102 S103 S104 S105 L9 S106 S107 S108 S109 S110 S111 S112 S113 S114 S115 S116 L10 S117 S118 S119 S120 S121 S122 S123 S124 S125 S126 S127 S128 S129 S130 L11 S131 S132 S133 S134 L12 S135 S136 S137 S138 S139 S140 S141 L13 S142 S143 S144 S145 S146 S147 S148 S149 S150 S151 S152 S153 S154 S155 S156 L14 S157 L15 S158 L16 S159 S160 S161 S162 S163 S164 S165 S166 S167 S168 L17 S169 S170 S171 S172 S173 L18 L19 S174 S175 S176 S177 S178 | L20 L21 L22 L23 | L28 L29 L30 L31 bodies 16 17 18 19 20
extrude "Extrude5" add sketch "Sketch4" against normal blind 1 contours L28 L29 L30 L31 bodies 16
fillet "Fillet1" radius 8.5 4 edges at (213.8586, 29.9009, 0.5) (213.8586, -6.0554, 0.5) (286.7595, -6.0554, 0.5) (286.7595, 29.9009, 0.5) on bodies 16
fillet "Fillet2" radius 9.5 4 edges at (287.7595, 30.9009, 0.3) (287.7595, -7.0554, 0.3) (212.8586, 30.9009, 0.3) (212.8586, -7.0554, 0.3) on bodies 16
